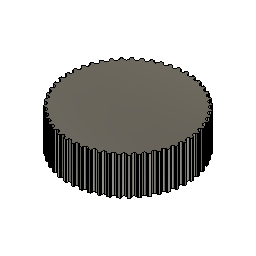
gear_51z (Autodesk Fusion 360 design; units mm, degrees)
Autodesk Fusion 360 part; units mm, degrees
sketch "Sketch1" plane through (0, 0, 0) normal (0, 0, 1) x (1, 0, 0) in component "gt2 pulley"
  circle A0 centre (0, 0) radius 16.2338 construction
  circle A1 centre (0, 0) radius 15.2298 construction
  line L0 (0, 0) -> (0, 16.2338) construction
  line L1 (0, 0) -> (0.9994, 16.203) construction
  line L2 (0, 0) -> (1.4071, 16.1727) construction
  circle A2 centre (0, 0) radius 15.9798 construction
  arc A3 (0.3883, 15.84) -> (0.4562, 15.5493) centre (1.3851, 15.9197) ccw
  circle A4 centre (0, 0) radius 15.8298 construction
  arc A5 (0.2409, 15.978) -> (0, 15.9798) centre (0, 0) ccw
  arc A6 (0.3883, 15.84) -> (0.2409, 15.978) centre (0.2387, 15.828) ccw
  arc A7 (0.4562, 15.5493) -> (0.9376, 15.2009) centre (0.9717, 15.7549) ccw
  arc A8 (0, 15.9798) -> (-0.2409, 15.978) centre (0, 0) ccw
  arc A9 (-0.2409, 15.978) -> (-0.3883, 15.84) centre (-0.2387, 15.828) ccw
  arc A10 (-0.4562, 15.5493) -> (-0.3883, 15.84) centre (-1.3851, 15.9197) ccw
  arc A11 (-0.9376, 15.2009) -> (-0.4562, 15.5493) centre (-0.9717, 15.7549) ccw
  arc A12 (0.9376, 15.2009) -> (-0.9376, 15.2009) centre (0, 0) ccw
  point P0 (1.3851, 15.9197)
  point P1 (0, 15.9798)
  dimension "d18" = 32.4676
  dimension "d19" = 3.529
  dimension "d22" = 1.004
  dimension "d24" = 0.75
  dimension "d26" = 1
  dimension "d27" = 0.15
  dimension "d28" = 0.15
  dimension "d47" = 0.555
  dimension "d52" = 3.812
  constraint coincident A0.centre A1.centre
  constraint coincident A0 L0.end
  constraint vertical L0
  constraint coincident A0 L1.end
  constraint coincident A0 L2.end
  constraint concentric A1 A2
  constraint coincident A1 A7.end
  constraint coincident L1 A7.end
  constraint coincident A2 P0
  constraint coincident L2 P0
  constraint coincident P0 A3.centre
  constraint coincident A2 P1
  constraint coincident L0 P1
  constraint concentric A2 A4
  constraint coincident P1 A5.end
  constraint coincident A4 A6.centre
  constraint coincident A3.start A6.start
  constraint tangent A3 A6
  constraint tangent A3 A7
  constraint symmetric L0 A7.end A11.start
  constraint symmetric L0 A3.start A9.end
  constraint symmetric L0 A3.end A10.start
  constraint symmetric L0 A3 A10
  constraint symmetric L0 A5.start A8.end
  constraint symmetric L0 P1 A5.end
  constraint symmetric L0 A5 A8
  constraint symmetric L0 A6 A9
  constraint symmetric L0 A7 A11
  constraint coincident A1 A11.start
  constraint tangent A1 A7
  constraint coincident L1 A7.centre
  measures "d18" diameter of A0
  measures "d19" angle of L0 L1
  measures "d22" distance of A0 A1
  measures "d24" distance of A1 A2
  measures "d26" radius of A3
  measures "d27" distance of A2 A4
  measures "d28" radius of A6
  measures "d47" radius of A7
extrude "Extrude1" add sketch "Sketch1" along normal blind 10 makes body 1
pattern_circular "C-Pattern1" count 51 over 360 about axis through (0, 0, 1.75) along (0, 0, 1) of bodies 1 makes body 2 at (-2.5933, 15.0074, 6.6667) makes body 3 at (-3.8158, 14.744, 6.6667) makes body 4 at (-6.1755, 13.9216, 6.6667) makes body 5 at (-7.2968, 13.368, 6.6667) makes body 6 at (-8.194, 12.8377, 3.3333) makes body 7 at (-9.7094, 11.7334, 3.3333) makes body 8 at (-11.4975, 9.9877, 3.3333) makes body 9 at (-12.2781, 9.0108, 3.3333) makes body 10 at (-13.2924, 7.4336, 3.3333) makes body 11 at (-14.1052, 5.7438, 3.3333) makes body 12 at (-14.8992, 3.1563, 6.6667) makes body 13 at (-15.1741, 1.3014, 6.6667) makes body 14 at (-15.2276, 0.2606, 3.3333) makes body 15 at (-15.1442, -1.6127, 3.3333) makes body 16 at (-14.8312, -3.4615, 3.3333) makes body 17 at (-14.2934, -5.2578, 3.3333) makes body 18 at (-13.539, -6.9745, 3.3333) makes body 19 at (-11.7001, -9.7496, 6.6667) makes body 20 at (-10.4133, -11.1135, 6.6667) makes body 21 at (-10.1052, -11.3944, 3.3333) makes body 22 at (-7.9286, -13.0032, 6.6667) makes body 23 at (-7.0208, -13.515, 3.3333) makes body 24 at (-5.3067, -14.2753, 3.3333) makes body 25 at (-3.5122, -14.8193, 3.3333) makes body 26 at (-0.8335, -15.207, 6.6667) makes body 27 at (1.0416, -15.1941, 6.6667) makes body 28 at (2.9009, -14.951, 6.6667) makes body 29 at (4.7162, -14.4812, 6.6667) makes body 30 at (7.0208, -13.515, 6.6667) makes body 31 at (7.3881, -13.3178, 3.3333) makes body 32 at (9.6289, -11.7996, 6.6667) makes body 33 at (11.4289, -10.0662, 6.6667) makes body 34 at (11.7001, -9.7495, 3.3333) makes body 35 at (13.2412, -7.5244, 6.6667) makes body 36 at (13.7248, -6.6013, 3.3333) makes body 37 at (14.432, -4.8646, 3.3333) makes body 38 at (15.0652, -2.2331, 6.6667) makes body 39 at (15.2254, -0.3648, 6.6667) makes body 40 at (15.1549, 1.509, 6.6667) makes body 41 at (14.8546, 3.3599, 6.6667) makes body 42 at (14.59, 4.368, 3.3333) makes body 43 at (13.9426, 6.1278, 3.3333) makes body 44 at (13.0839, 7.7947, 3.3333) makes body 45 at (12.0269, 9.3435, 3.3333) makes body 46 at (10.7875, 10.7507, 3.3333) makes body 47 at (9.3846, 11.9948, 3.3333) makes body 48 at (7.1131, 13.4666, 6.6667) makes body 49 at (5.4043, 14.2387, 6.6667) makes body 50 at (3.0031, 14.9308, 6.6667) makes body 51 at (1.7681, 15.1268, 6.6667)
sketch "Sketch2" plane through (0, 0, 10) normal (0, 0, 1) x (-1, 0, 0)
  arc A0 (-7.8359, -13.7715) -> (-7.7714, -13.9628) centre (-7.6985, -13.8317) ccw
  arc A1 (-7.7714, -13.9628) -> (-7.3468, -14.1908) centre (0, 0) ccw
  arc A2 (-7.3468, -14.1908) -> (-7.1517, -14.1389) centre (-7.2778, -14.0576) ccw
  arc A3 (-6.9544, -13.915) -> (-7.1517, -14.1389) centre (-6.3112, -14.6807) ccw
  arc A4 (-6.3655, -13.8357) -> (-6.9544, -13.915) centre (-6.5974, -14.3399) ccw
  arc A5 (-8.0175, -12.9486) -> (-6.3655, -13.8357) centre (0, 0) ccw
  arc A6 (-7.7582, -13.4833) -> (-8.0175, -12.9486) centre (-8.3096, -13.4205) ccw
  arc A7 (-7.8359, -13.7715) -> (-7.7582, -13.4833) centre (-8.7518, -13.3701) ccw
  circle A8 centre (0, 0) radius 15.2298
  constraint concentric A1 A8
extrude "Extrude2" add sketch "Sketch2" against normal blind 10 contours A5 A8 bodies 1 2 3 4 5 6 7 8 9 10 11 12 13 14 15 16 17 18 19 20 21 22 23 24 25 26 27 28 29 30 31 32 33 34 35 36 37 38 39 40 41 42 43 44 45 46 47 48 49 50 51
extrude "Extrude4" [suppressed] in component "gt2 pulley"
pattern_circular "C-Pattern7" [suppressed] in component "gt2 pulley"
extrude "Extrude3" [suppressed] in component "gt2 pulley"
pattern_circular "C-Pattern6" [suppressed] in component "gt2 pulley"
extrude "Extrude2'" [suppressed] in component "gt2 pulley"
pattern_circular "C-Pattern5" [suppressed] in component "gt2 pulley"
extrude "Extrude1'" [suppressed] in component "gt2 pulley"
pattern_circular "C-Pattern4" [suppressed] in component "gt2 pulley"
pattern_circular "C-Pattern3" [suppressed] in component "gt2 pulley"
pattern_circular "C-Pattern2" [suppressed] in component "gt2 pulley"
pattern_circular "C-Pattern1'" [suppressed] in component "gt2 pulley"
copy_body "Body->Comp1" [suppressed] in component "Component"
copy_body "Body->Comp2" [suppressed] in component "Component'"
copy_body "Body->Comp3" [suppressed] in component "Component''"
copy_body "Body->Comp4" [suppressed] in component "Component'''"
copy_body "Body->Comp5" [suppressed] in component "Component''''"
copy_body "Body->Comp6" [suppressed] in component "Component'''''"
copy_body "Body->Comp7" [suppressed] in component "Component''''''"
copy_body "Body->Comp8" [suppressed] in component "Component'''''''"
copy_body "Body->Comp9" [suppressed] in component "Component''''''''"
copy_body "Body->Comp10" [suppressed] in component "Component'''''''''"
copy_body "Body->Comp11" [suppressed] in component "Component''''''''''"
copy_body "Body->Comp12" [suppressed] in component "Component'''''''''''"
copy_body "Body->Comp13" [suppressed] in component "Component''''''''''''"
copy_body "Body->Comp14" [suppressed] in component "Component'''''''''''''"
copy_body "Body->Comp15" [suppressed] in component "Component''''''''''''''"
copy_body "Body->Comp16" [suppressed] in component "Component'''''''''''''''"
copy_body "Body->Comp17" [suppressed] in component "Component''''''''''''''''"
copy_body "Body->Comp18" [suppressed] in component "Component'''''''''''''''''"
copy_body "Body->Comp19" [suppressed] in component "Component''''''''''''''''''"
copy_body "Body->Comp20" [suppressed] in component "Component'''''''''''''''''''"
component "gt2 pulley" placed x (1, 0, 0) y (0, 1, 0) z (0, 0, 1) at (0, 0, 0)
equation "NumTeeth = 51" comment "min 20"
equation "ToothPitch = 2 mm"
equation "PullyDia = NumTeeth * ToothPitch / PI"
equation "ToothAng = ( ( 360 / NumTeeth ) * 1 deg )"
equation "TransOffsetAngle = ToothAng * 0.2"
equation "Sholulder_Radius = 0.15 mm"
equation "Root_Radius = 0.555 mm"
equation "TransRadius = 1 mm"
equation "ToolHeight = 0.75 mm"
equation "PLD = 0.254 mm"
equation "d18 = PullyDia"
equation "d19 = ToothAng / 2"
equation "d22 = PLD + ToolHeight"
equation "d24 = ToolHeight"
equation "d26 = TransRadius"
equation "d27 = Sholulder_Radius"
equation "d31 = NumTeeth"
equation "d33 = NumTeeth"
equation "d35 = NumTeeth"
equation "d37 = NumTeeth"
equation "d41 = NumTeeth"
equation "d45 = NumTeeth"
equation "d47 = Root_Radius"
equation "d50 = NumTeeth"
